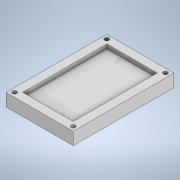
# Autodesk Inventor part: Water_Proof_Box_Top
Saved by Autodesk Inventor 2022 (Build 260153000, 153)
## iProperties
Created: 2023-07-12
Part Number: Water_Proof_Box_Top
Material: Generic
Document SubType Name: Modeling
Designer: jtw4137
Density: 1 g/cm^3
Appearance: Default
Author: jtw4137
Autodesk Inventor part; units mm, degrees
ref_plane "YZ Plane" through (0, 0, 0) normal (1, 0, 0) x (0, 1, 0)
ref_plane "XZ Plane" through (0, 0, 0) normal (0, 1, 0) x (-1, 0, 0)
ref_plane "XY Plane" through (0, 0, 0) normal (0, 0, 1) x (1, 0, 0)
sketch "Sketch1" plane through (0, 0, 0) normal (0, 1, 0) x (-1, 0, 0)
  line L0 (0, 0) -> (80, 0)
  line L1 (80, 0) -> (80, -120)
  line L2 (80, -120) -> (0, -120)
  line L3 (0, -120) -> (0, 0)
  dimension "d0" = 120
  dimension "d1" = 80
  constraints: 8 end point, 3 perpendicular
  measures "d0" distance of L0.end L1.end
  measures "d1" distance of L0.start L0.end
extrude "Extrusion1" add sketch "Sketch1" along normal blind 15
shell "Shell1" thickness 10 removed faces 1 at (-26.6667, 15, -80)
sketch "Sketch3" plane through (0, 15, 0) normal (0, 1, 0) x (1, 0, 0)
  line L0 (-80, 0) -> (0, 0) projected
  line L1 (0, 0) -> (0, 4.953)
  line L2 (0, 0) -> (0, 120) projected
  line L3 (-4.953, 4.953) -> (0, 4.953)
  line L4 (-4.953, 4.953) -> (-4.953, 0)
  dimension "d5" = 4.953
  dimension "d6" = 4.953
  constraints: 6 end point, 1 perpendicular, 1 point on line, 1 vertical
  measures "d5" distance of L3.start L4.end
  measures "d6" distance of L3.start L1.end
hole "Hole1" at (-4.953, 15, -4.953) direction (0, -1, 0) diameter 5 end through all
sketch "Sketch5" plane through (0, 15, 0) normal (0, 1, 0) x (1, 0, 0)
  line L0 (-70, 10) -> (-70, 110) projected
  line L1 (-70, 10) -> (-74.953, 10)
  line L2 (-74.953, 10) -> (-74.953, 5.047)
  point P0 (0, 0)
  dimension "d14" = 4.953
  dimension "d15" = 4.953
  constraints: 4 end point, 1 horizontal, 1 perpendicular
  measures "d14" distance of L0.start L1.end
  measures "d15" distance of L1.end L2.end
hole "Hole2" at (-74.953, 15, -5.047) direction (0, -1, 0) diameter 5 end through all
sketch "Sketch6" plane through (0, 15, 0) normal (0, 1, 0) x (1, 0, 0)
  line L0 (-70, 110) -> (-10, 110) projected
  line L1 (-70, 110) -> (-70, 114.953)
  line L2 (-70, 114.953) -> (-74.953, 114.953)
  point P0 (0, 0)
  dimension "d23" = 4.953
  dimension "d24" = 4.953
  constraints: 4 end point, 1 perpendicular, 1 vertical
  measures "d23" distance of L0.start L1.end
  measures "d24" distance of L1.end L2.end
hole "Hole3" at (-74.953, 15, -114.953) direction (0, -1, 0) diameter 5 end through all
sketch "Sketch7" plane through (0, 15, 0) normal (0, 1, 0) x (1, 0, 0)
  line L0 (-70, 110) -> (-10, 110) projected
  line L1 (-10, 110) -> (-10, 114.953)
  line L2 (-10, 114.953) -> (-5.047, 114.953)
  point P0 (0, 0)
  dimension "d32" = 4.953
  dimension "d33" = 4.953
  constraints: 4 end point, 1 perpendicular, 1 vertical
  measures "d32" distance of L0.end L1.end
  measures "d33" distance of L1.end L2.end
hole "Hole4" at (-5.047, 15, -114.953) direction (0, -1, 0) diameter 5 end through all
body "Solid1"
